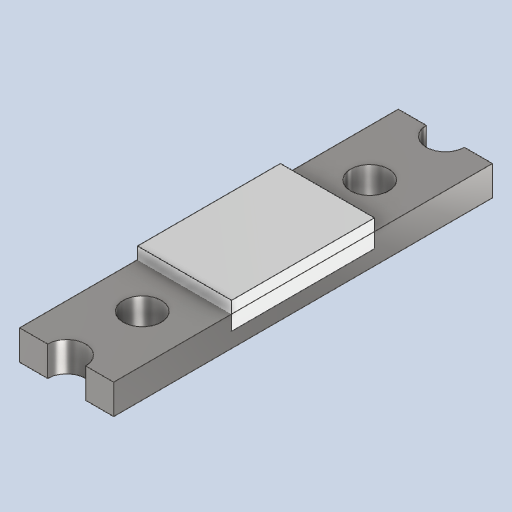
# Autodesk Inventor part: SC700-40kg
Saved by Autodesk Inventor 2022.3 (Build 263350000, 350)
## iProperties
Part Number: SC700-40kg
Material: Generic
Document SubType Name: Modeling
Designer: Masato Kubotera
Density: 1 g/cm^3
Appearance: Default
Catalog Web Link: https://www.alibaba.com/product-detail/SC700-Luggage-Scale-Weight-Sensor-Miniature_60710753448.html
Author: Masato Kubotera
Autodesk Inventor part; units mm, degrees
ref_plane "YZ Plane" through (0, 0, 0) normal (1, 0, 0) x (0, 1, 0)
ref_plane "XZ Plane" through (0, 0, 0) normal (0, 1, 0) x (-1, 0, 0)
ref_plane "XY Plane" through (0, 0, 0) normal (0, 0, 1) x (1, 0, 0)
sketch "Sketch1" plane through (0, 0, 0) normal (0, 0, 1) x (1, 0, 0)
  line L0 (-15.9, -3.95) -> (15.9, -3.95)
  line L1 (15.9, -3.95) -> (15.9, 3.95)
  line L2 (15.9, 3.95) -> (-15.9, 3.95)
  line L3 (-15.9, 3.95) -> (-15.9, -3.95)
  line L4 (-15.9, -3.95) -> (15.9, 3.95) construction
  line L5 (15.9, -3.95) -> (-15.9, 3.95) construction
  line L6 (-15.9, 0) -> (15.9, 0) construction
  line L7 (0, 3.95) -> (0, -3.95) construction
  circle A0 centre (9.55, 0) radius 1.6
  arc A1 (15.9, 1.6) -> (15.9, -1.6) centre (15.9, 0) ccw
  circle A2 centre (-9.55, 0) radius 1.6
  arc A3 (-15.9, -1.6) -> (-15.9, 1.6) centre (-15.9, 0) ccw
  line L8 (6, 3.95) -> (6, -3.95)
  line L9 (-6, 3.95) -> (-6, -3.95)
  point P0 (0, 0)
  point P1 (-15.9, 1.6)
  point P2 (-15.9, -1.6)
  dimension "d0" = 31.8
  dimension "d1" = 7.9
  dimension "d2" = 3.2
  dimension "d3" = 19.1
  dimension "d4" = 12
  constraints: 20 end point, 6 midpoint, 6 symmetric about line, 5 point on line, 4 centre point, 4 point on circle, 2 parallel, 2 perpendicular, 1 coincident, 1 equal radius, 1 horizontal, 2 other
  measures "d0" distance of L1.end L2.end
  measures "d1" distance of L2.end L0.start
  measures "d2" diameter of A0
  measures "d3" distance of A0.centre A2.centre
  measures "d4" distance between parallel lines of L8 L9
extrude "Extrusion1" add sketch "Sketch1" along normal mid plane 2.5 contours L3 A3 L2 L9 L0 | L9 L2 L8 L0 | L8 L2 L1 A1 L0
extrude "Extrusion2" add sketch "Sketch1" along normal blind 2.25 separate body contours L9 L2 L8 L0
body "Solid1"
